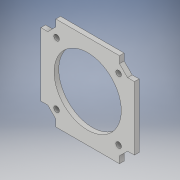
# Autodesk Inventor part: LC_lens_holder_outer
Saved by Autodesk Inventor 2019 (Build 230136000, 136)
## iProperties
Created: 2021-05-17
Part Number: LC_lens_holder_outer
Material: Generic
Document SubType Name: Modeling
Designer: UC2
Density: 1 g/cm^3
Appearance: Default
Author: UC2
Autodesk Inventor part; units mm, degrees
ref_plane "YZ Plane" through (0, 0, 0) normal (1, 0, 0) x (0, 1, 0)
ref_plane "XZ Plane" through (0, 0, 0) normal (0, 1, 0) x (-1, 0, 0)
ref_plane "XY Plane" through (0, 0, 0) normal (0, 0, 1) x (1, 0, 0)
sketch "Skizze1" plane through (0, 0, 0) normal (0, 0, 1) x (1, 0, 0)
  line L0 (-37.707, 0) -> (50.8634, 0) construction
  line L1 (0, -35.4687) -> (0, 37.4335) construction
  line L2 (0, 0) -> (27.0189, 27.0189) construction
  line L3 (0, 0) -> (38.2105, 0) construction
  line L4 (0, 24.9041) -> (16.9, 24.9041)
  line L5 (16.9, 24.9041) -> (16.9, 21.2841)
  line L6 (16.9, 21.2841) -> (19.092, 19.092)
  line L7 (24.9041, 0) -> (24.9041, 16.9)
  line L8 (24.9041, 16.9) -> (21.2841, 16.9)
  line L9 (21.2841, 16.9) -> (19.092, 19.092)
  line L10 (0, 24.9041) -> (-16.9, 24.9041)
  line L11 (-16.9, 24.9041) -> (-16.9, 21.2841)
  line L12 (-16.9, 21.2841) -> (-19.092, 19.092)
  line L13 (-24.9041, 0) -> (-24.9041, 16.9)
  line L14 (-24.9041, 16.9) -> (-21.2841, 16.9)
  line L15 (-21.2841, 16.9) -> (-19.092, 19.092)
  line L16 (0, -24.9041) -> (16.9, -24.9041)
  line L17 (16.9, -24.9041) -> (16.9, -21.2841)
  line L18 (16.9, -21.2841) -> (19.092, -19.092)
  line L19 (24.9041, 0) -> (24.9041, -16.9)
  line L20 (24.9041, -16.9) -> (21.2841, -16.9)
  line L21 (21.2841, -16.9) -> (19.092, -19.092)
  line L22 (0, -24.9041) -> (-16.9, -24.9041)
  line L23 (-16.9, -24.9041) -> (-16.9, -21.2841)
  line L24 (-16.9, -21.2841) -> (-19.092, -19.092)
  line L25 (-24.9041, 0) -> (-24.9041, -16.9)
  line L26 (-24.9041, -16.9) -> (-21.2841, -16.9)
  line L27 (-21.2841, -16.9) -> (-19.092, -19.092)
  circle A0 centre (0, 0) radius 18
  circle A1 centre (-16.6172, 16.6172) radius 1.5
  line L28 (-16.6172, 16.6172) -> (16.6172, 16.6172) construction
  line L29 (16.6172, 16.6172) -> (16.6172, -16.6172) construction
  line L30 (16.6172, -16.6172) -> (-16.6172, -16.6172) construction
  line L31 (-16.6172, -16.6172) -> (-16.6172, 16.6172) construction
  circle A2 centre (16.6172, 16.6172) radius 1.5
  circle A3 centre (-16.6172, -16.6172) radius 1.5
  circle A4 centre (16.6172, -16.6172) radius 1.5
  line L32 (-17.05, 25.0541) -> (0, 25.0541)
  line L33 (0, 25.0541) -> (17.05, 25.0541)
  line L34 (17.05, 25.0541) -> (17.05, 21.3462)
  line L35 (17.05, 21.3462) -> (19.1981, 19.1981)
  line L36 (19.1981, 19.1981) -> (21.3462, 17.05)
  line L37 (21.3462, 17.05) -> (25.0541, 17.05)
  line L38 (25.0541, 17.05) -> (25.0541, 0)
  line L39 (25.0541, 0) -> (25.0541, -17.05)
  line L40 (25.0541, -17.05) -> (21.3462, -17.05)
  line L41 (21.3462, -17.05) -> (19.1981, -19.1981)
  line L42 (19.1981, -19.1981) -> (17.05, -21.3462)
  line L43 (17.05, -21.3462) -> (17.05, -25.0541)
  line L44 (17.05, -25.0541) -> (0, -25.0541)
  line L45 (0, -25.0541) -> (-17.05, -25.0541)
  line L46 (-17.05, -25.0541) -> (-17.05, -21.3462)
  line L47 (-17.05, -21.3462) -> (-19.1981, -19.1981)
  line L48 (-19.1981, -19.1981) -> (-21.3462, -17.05)
  line L49 (-21.3462, -17.05) -> (-25.0541, -17.05)
  line L50 (-25.0541, -17.05) -> (-25.0541, 0)
  line L51 (-25.0541, 0) -> (-25.0541, 17.05)
  line L52 (-25.0541, 17.05) -> (-21.3462, 17.05)
  line L53 (-21.3462, 17.05) -> (-19.1981, 19.1981)
  line L54 (-19.1981, 19.1981) -> (-17.05, 21.3462)
  line L55 (-17.05, 21.3462) -> (-17.05, 25.0541)
  dimension "d0" = 45
  dimension "d1" = 16.9
  dimension "d2" = 3.62
  dimension "d3" = 3.1
  dimension "d4" = 36
  dimension "d7" = 3
  dimension "d8" = 3
  dimension "d9" = 3
  dimension "d10" = 3
  dimension "d11" = 3.5
  dimension "d12" = 0.15
  constraints: 108 end point, 20 symmetric about line, 5 centre point, 5 coincident, 4 perpendicular, 4 point on line, 3 horizontal, 2 parallel, 1 equal length, 24 other
  measures "d0" angle of L3 L2
  measures "d1" distance of L4.start L4.end
  measures "d2" distance of L4.end L5.end
  measures "d3" distance of L5.end L6.end
  measures "d4" diameter of A0
  measures "d7" diameter of A1
  measures "d8" diameter of A2
  measures "d9" diameter of A3
  measures "d10" diameter of A4
  measures "d11" distance of L6.end A2.centre
  measures "d12" distance between parallel lines of L10 L32
extrude "Extrusion1" add sketch "Skizze1" along normal blind 2.5 contours L4 L5 L6 L9 L8 L7 L19 L20 L21 L18 L17 L16 L22 L23 L24 L27 L26 L25 L13 L14 L15 L12 L11 L10 | L32 L33 L34 L35 L36 L37 L38 L39 L40 L41 L42 L43 L44 L45 L46 L47 L48 L49 L50 L51 L52 L53 L54 L55
equation "\"d8\" = d7"
equation "\"d9\" = d7"
equation "\"d10\" = d7"
